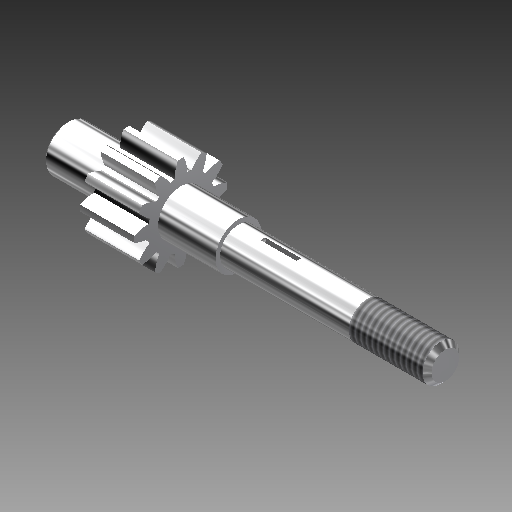
# Autodesk Inventor part: Shaft
Saved by Autodesk Inventor 2020 (Build 240168000, 168)
## iProperties
CustomPartVersion: 1
Created: 2016-04-28
Part Number: Shaft
Material: Aluminum 6061
Document SubType Name: Modeling
Designer: Jorge
Density: 2.7 g/cm^3
Appearance: Aluminum - Flat
Mass: 76.5537 g
Surface Area: 92.3728 cm^2
Volume: 28.3532 cm^3
Author: Jorge
Autodesk Inventor part; units mm, degrees
ref_plane "Start Plane" through (0, 0, 0) normal (1, 0, 0) x (0, 1, 0)
ref_plane "XZ Plane" through (0, 0, 0) normal (0, 1, 0) x (-1, 0, 0)
ref_plane "XY Plane" through (0, 0, 0) normal (0, 0, 1) x (1, 0, 0)
sketch "Main Sketch" plane through (0, 0, 0) normal (0, 0, 1) x (1, 0, 0)
  line L0 (0, 0) -> (130.7338, 0)
  line L1 (0, 0) -> (0, 7.9216)
  line L2 (0, 7.9216) -> (20.6375, 7.9216)
  line L3 (20.6375, 7.9216) -> (20.6375, 11.3284)
  line L4 (39.4335, 11.3284) -> (39.4335, 7.9216)
  line L5 (20.6375, 11.3284) -> (39.4335, 11.3284)
  line L6 (59.2963, 7.9216) -> (59.2963, 6.35)
  line L7 (39.4335, 7.9216) -> (59.2963, 7.9216)
  line L8 (130.7338, 6.35) -> (130.7338, 0)
  line L9 (59.2963, 6.35) -> (130.7338, 6.35)
  dimension "d3" = 15.8432
  dimension "d4" = 22.6568
  dimension "d5" = 15.8432
  dimension "d6" = 12.7
  constraints: 20 end point, 5 horizontal, 5 vertical
  measures "d3" diameter of L2 L0
  measures "d4" diameter of L5 L0
  measures "d5" diameter of L7 L0
  measures "d6" diameter of L9 L0
revolve "Revolution1" add sketch "Main Sketch" angle 360 about axis through (0, 0, 0) along (1, 0, 0)
chamfer "Chamfer1" distance 0.7937 angle 45 1 edges at (0, -7.9216, 0) measured on face at (13.7583, 7.8959, -0.6374)
chamfer "Chamfer2" distance 1.5875 angle 45 1 edges at (130.7338, -6.35, 0) measured on face at (106.9213, 6.2678, -1.0186)
thread "Thread1" size "1/2-13 UNC" class "2A" standard "ANSI Unified Screw Threads" length 25.4
sketch "Sketch3" plane through (0, 0, 0) normal (0, 0, 1) x (1, 0, 0)
  arc A0 (67.6045, 7.4481) -> (80.2341, 7.4481) centre (73.9193, 7.4481) ccw
  line L0 (67.6045, 7.4481) -> (80.2341, 7.4481)
  line L1 (59.2963, -7.9216) -> (59.2963, 7.9216) construction
  point P0 (0, 0)
  dimension "d16" = 14.623
  dimension "d17" = 6.3148
  constraints: 2 end point, 2 point on circle, 1 centre point, 1 horizontal
  measures "d16" distance from line of A0.centre L1
  measures "d17" radius of A0
extrude "Extrusion1" cut sketch "Sketch3" along normal mid plane 1.5875
sketch "Sketch4" plane through (39.4335, 0, 0) normal (1, 0, 0) x (0, 0, -1)
  arc A0 (-8.9345, 13.3715) -> (-7.4665, 8.514) centre (3.948, 14.6141) ccw
  arc A1 (-7.4665, 8.514) -> (-8.514, 7.4665) centre (0, 0) ccw
  arc A2 (-8.514, 7.4665) -> (-13.3715, 8.9345) centre (-14.6141, -3.948) ccw
  arc A3 (-13.3715, 8.9345) -> (-14.4233, 7.1128) centre (0, 0) ccw
  arc A4 (-14.4233, 7.1128) -> (-10.7232, 3.64) centre (-3.888, 14.6302) ccw
  arc A5 (-10.7232, 3.64) -> (-11.1066, 2.2092) centre (0, 0) ccw
  arc A6 (-11.1066, 2.2092) -> (-16.0473, 1.0518) centre (-10.6822, -10.7261) ccw
  arc A7 (-16.0473, 1.0518) -> (-16.0473, -1.0518) centre (0, 0) ccw
  arc A8 (-16.0473, -1.0518) -> (-11.1066, -2.2092) centre (-10.6822, 10.7261) ccw
  arc A9 (-11.1066, -2.2092) -> (-10.7232, -3.64) centre (0, 0) ccw
  arc A10 (-10.7232, -3.64) -> (-14.4233, -7.1128) centre (-3.888, -14.6302) ccw
  arc A11 (-14.4233, -7.1128) -> (-13.3715, -8.9345) centre (0, 0) ccw
  arc A12 (-13.3715, -8.9345) -> (-8.514, -7.4665) centre (-14.6141, 3.948) ccw
  arc A13 (-8.514, -7.4665) -> (-7.4665, -8.514) centre (0, 0) ccw
  arc A14 (-7.4665, -8.514) -> (-8.9345, -13.3715) centre (3.948, -14.6141) ccw
  arc A15 (-8.9345, -13.3715) -> (-7.1128, -14.4233) centre (0, 0) ccw
  arc A16 (-7.1128, -14.4233) -> (-3.64, -10.7232) centre (-14.6302, -3.888) ccw
  arc A17 (-3.64, -10.7232) -> (-2.2092, -11.1066) centre (0, 0) ccw
  arc A18 (-2.2092, -11.1066) -> (-1.0518, -16.0473) centre (10.7261, -10.6822) ccw
  arc A19 (-1.0518, -16.0473) -> (1.0518, -16.0473) centre (0, 0) ccw
  arc A20 (1.0518, -16.0473) -> (2.2092, -11.1066) centre (-10.7261, -10.6822) ccw
  arc A21 (2.2092, -11.1066) -> (3.64, -10.7232) centre (0, 0) ccw
  arc A22 (3.64, -10.7232) -> (7.1128, -14.4233) centre (14.6302, -3.888) ccw
  arc A23 (7.1128, -14.4233) -> (8.9345, -13.3715) centre (0, 0) ccw
  arc A24 (8.9345, -13.3715) -> (7.4665, -8.514) centre (-3.948, -14.6141) ccw
  arc A25 (7.4665, -8.514) -> (8.514, -7.4665) centre (0, 0) ccw
  arc A26 (8.514, -7.4665) -> (13.3715, -8.9345) centre (14.6141, 3.948) ccw
  arc A27 (13.3715, -8.9345) -> (14.4233, -7.1128) centre (0, 0) ccw
  arc A28 (14.4233, -7.1128) -> (10.7232, -3.64) centre (3.888, -14.6302) ccw
  arc A29 (10.7232, -3.64) -> (11.1066, -2.2092) centre (0, 0) ccw
  arc A30 (11.1066, -2.2092) -> (16.0473, -1.0518) centre (10.6822, 10.7261) ccw
  arc A31 (16.0473, -1.0518) -> (16.0473, 1.0518) centre (0, 0) ccw
  arc A32 (16.0473, 1.0518) -> (11.1066, 2.2092) centre (10.6822, -10.7261) ccw
  arc A33 (11.1066, 2.2092) -> (10.7232, 3.64) centre (0, 0) ccw
  arc A34 (10.7232, 3.64) -> (14.4233, 7.1128) centre (3.888, 14.6302) ccw
  arc A35 (14.4233, 7.1128) -> (13.3715, 8.9345) centre (0, 0) ccw
  arc A36 (13.3715, 8.9345) -> (8.514, 7.4665) centre (14.6141, -3.948) ccw
  arc A37 (8.514, 7.4665) -> (7.4665, 8.514) centre (0, 0) ccw
  arc A38 (7.4665, 8.514) -> (8.9345, 13.3715) centre (-3.948, 14.6141) ccw
  arc A39 (8.9345, 13.3715) -> (7.1128, 14.4233) centre (0, 0) ccw
  arc A40 (7.1128, 14.4233) -> (3.64, 10.7232) centre (14.6302, 3.888) ccw
  arc A41 (3.64, 10.7232) -> (2.2092, 11.1066) centre (0, 0) ccw
  arc A42 (2.2092, 11.1066) -> (1.0518, 16.0473) centre (-10.7261, 10.6822) ccw
  arc A43 (1.0518, 16.0473) -> (-1.0518, 16.0473) centre (0, 0) ccw
  arc A44 (-1.0518, 16.0473) -> (-2.2092, 11.1066) centre (10.7261, 10.6822) ccw
  arc A45 (-2.2092, 11.1066) -> (-3.64, 10.7232) centre (0, 0) ccw
  arc A46 (-3.64, 10.7232) -> (-7.1128, 14.4233) centre (-14.6302, 3.888) ccw
  arc A47 (-7.1128, 14.4233) -> (-8.9345, 13.3715) centre (0, 0) ccw
  constraints: 96 point on circle, 48 centre point
extrude "Extrusion2" add sketch "Sketch4" against normal up to surface (18.796 mm away)
body "Solid1"
